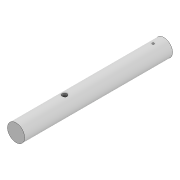
# Autodesk Inventor part: Barra_circular_soporte
Saved by Autodesk Inventor 2021 (Build 250183000, 183)
## iProperties
Created: 2021-04-16
Part Number: Barra_circular_soporte
Material: Genérico
Document SubType Name: Modeling
Designer: Admin
Density: 1 g/cm^3
Appearance: Valor por defecto
Author: Admin
Autodesk Inventor part; units mm, degrees
ref_plane "YZ Plane" through (0, 0, 0) normal (1, 0, 0) x (0, 1, 0)
ref_plane "XZ Plane" through (0, 0, 0) normal (0, 1, 0) x (-1, 0, 0)
sketch "Boceto1" plane through (0, 0, 0) normal (0, 0, 1) x (1, 0, 0)
  circle A0 centre (0, 0) radius 8.73
  dimension "d0" = 17.46
  constraints: 1 centre point, 1 coincident
  measures "d0" diameter of A0
extrude "Extrusión1" add sketch "Boceto1" along normal blind 150
sketch "Boceto2" plane through (0, 0, 0) normal (0, 0, -1) x (-1, 0, 0)
  circle A0 centre (0, 0) radius 8.73 projected
  point P0 (0, 8.73)
  constraints: 1 vertical alignment, 1 other
ref_plane "Plano de trabajo1" through (0, 8.73, 0) normal (0, 1, 0) x (-1, 0, 0)
sketch "Boceto3" plane through (0, 8.73, 0) normal (0, 1, 0) x (-1, 0, 0)
  line L0 (0, 0) -> (0, 10.93)
  circle A0 centre (0, 10.93) radius 1
  circle A1 centre (0, 100.93) radius 2.5
  dimension "d3" = 10.93
  dimension "d4" = 2
  dimension "d7" = 5
  dimension "d8" = 90
  constraints: 2 centre point, 2 end point, 1 coincident, 1 vertical
  measures "d3" distance of L0.start L0.end
  measures "d4" diameter of A0
  measures "d7" diameter of A1
  measures "d8" distance of A1.centre L0.end
extrude "Extrusión2" cut sketch "Boceto3" against normal through all
